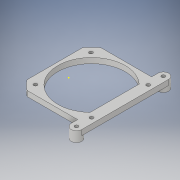
# Autodesk Inventor part: END
Saved by Autodesk Inventor 2019.4 (Build 234330000, 330)
## iProperties
Created: 2020-08-29
Part Number: END
Material: Generic
Document SubType Name: Modeling
Designer: craig
Density: 1 g/cm^3
Appearance: Default
Author: craig
## iProperties of the stored document _3DPrint.ipt
Created: 2020-08-29
Part Number: _3DPrint
Material: Generic
Document SubType Name: Modeling
Designer: craig
Density: 1 g/cm^3
Appearance: Default
Author: craig
Autodesk Inventor part; units mm, degrees
ref_plane "YZ Plane" through (0, 0, 0) normal (1, 0, 0) x (0, 1, 0)
ref_plane "XZ Plane" through (0, 0, 0) normal (0, 1, 0) x (-1, 0, 0)
ref_plane "XY Plane" through (0, 0, 0) normal (0, 0, 1) x (1, 0, 0)
sketch "Sketch1" plane through (0, 0, 0) normal (0, 1, 0) x (-1, 0, 0)
  line L0 (29, 24.5) -> (-29, 24.5) construction
  line L1 (-29, 24.5) -> (-29, -24.5) construction
  line L2 (-29, -24.5) -> (29, -24.5) construction
  line L3 (29, -24.5) -> (29, 24.5) construction
  line L4 (29, 24.5) -> (-29, -24.5) construction
  line L5 (-29, 24.5) -> (29, -24.5) construction
  circle A0 centre (29, 24.5) radius 1
  circle A1 centre (29, -24.5) radius 1
  circle A2 centre (-29, -24.5) radius 1
  circle A3 centre (-29, 24.5) radius 1
  circle A4 centre (29, 24.5) radius 3
  circle A5 centre (29, -24.5) radius 3
  circle A6 centre (-29, -24.5) radius 3
  circle A7 centre (-29, 24.5) radius 3
  point P0 (0, 0)
  dimension "d0" = 49
  dimension "d1" = 58
  dimension "d2" = 2
  dimension "d3" = 6
  constraints: 12 end point, 8 centre point, 8 coincident, 6 equal radius, 2 midpoint, 2 parallel, 1 horizontal, 1 perpendicular
  measures "d0" distance of L2.end L0.start
  measures "d1" distance of L0.start L0.end
  measures "d2" diameter of A0
  measures "d3" diameter of A4
extrude "Extrusion1" add sketch "Sketch1" along normal blind 5.8
sketch "Sketch2" plane through (-29, 5.8, 24.5) normal (0, 1, 0) x (1, 0, 0)
  line L0 (3, -0.001) -> (3, 48.999)
  line L1 (-3, 48.999) -> (-3, -0.001)
  circle A0 centre (0, 0) radius 1 projected
  line L2 (61, 0) -> (61, 49)
  line L3 (55, 49) -> (55, 0)
  circle A1 centre (58, 0) radius 1 projected
  circle A2 centre (0, 49) radius 1 projected
  circle A3 centre (58, 49) radius 1 projected
  line L4 (-3, -0.001) -> (-1, -0.001)
  line L5 (1, -0.001) -> (3, -0.001)
  line L6 (3, 48.999) -> (1, 48.999)
  line L7 (-1, 48.999) -> (-3, 48.999)
  line L8 (61, 49) -> (59, 49)
  line L9 (57, 49) -> (55, 49)
  line L10 (55, 0) -> (57, 0)
  line L11 (59, 0) -> (61, 0)
  point P0 (29, 24.5)
  dimension "d6" = 6
  dimension "d7" = 3
  dimension "d8" = 49
  dimension "d9" = 49
  dimension "d10" = 6
  dimension "d11" = 3
  constraints: 24 end point, 10 parallel, 8 point on circle, 4 horizontal, 4 perpendicular
  measures "d6" distance of L1.end L0.start
  measures "d7" distance from line of A0.centre L1
  measures "d8" distance of L1.start L1.end
  measures "d9" distance of L3.start L3.end
  measures "d10" distance of L3.end L2.start
  measures "d11" distance from line of A1.centre L3
extrude "Extrusion2" add sketch "Sketch2" against normal blind 3
sketch "Sketch3" plane through (-29, 2.8, 24.5) normal (0, -1, 0) x (1, 0, 0)
  circle A0 centre (0, -5) radius 2.5
  circle A1 centre (0, 0) radius 1 projected
  point P0 (29, -24.5)
  dimension "d14" = 5
  dimension "d15" = 5
  constraints: 1 centre point
  measures "d14" diameter of A0
  measures "d15" distance of A1.centre A0.centre
extrude "Extrusion3" cut sketch "Sketch3" against normal blind 2.8 contours A0
sketch "Sketch4" plane through (0, 5.8, 0) normal (0, 1, 0) x (1, 0, 0)
  circle A0 centre (29, -16) radius 1
  circle A1 centre (29, 16) radius 1
  circle A2 centre (29, -24.5) radius 1 projected
  point P0 (0, 0)
  dimension "d18" = 32
  dimension "d19" = 16
  dimension "d20" = 2
  dimension "d21" = 2
  dimension "d22" = 0
  constraints: 2 centre point, 1 vertical alignment
  measures "d18" distance of A1.centre A0.centre
  measures "d19" vertical distance of point (0, 0) A0.centre
  measures "d20" diameter of A0
  measures "d21" diameter of A1
  measures "d22" horizontal distance of A2.centre A0.centre
extrude "Extrusion4" cut sketch "Sketch4" against normal blind 2.8 contours A0 | A1
sketch "Sketch5" plane through (0, 5.8, 0) normal (0, 1, 0) x (1, 0, 0)
  line L0 (26, -24.5) -> (26, 24.5) projected
  circle A0 centre (-3, -15.6503) radius 0.9959
  circle A1 centre (29, -16) radius 1 projected
  arc A2 (-6, 0) -> (26, -13.8564) centre (13, 0) ccw
  arc A3 (-13, 0) -> (26, -22.5167) centre (13, 0) ccw
  line L1 (-13, 0) -> (-6, 0)
  point P0 (0, 0)
  dimension "d27" = 32
  dimension "d37" = 38
  dimension "d38" = 16
  dimension "d39" = 52
  constraints: 4 point on circle, 3 centre point, 2 end point, 2 point on line, 1 coincident
  measures "d27" horizontal distance of A1.centre A0.centre
  measures "d37" diameter of A2
  measures "d38" horizontal distance of A2.centre A0.centre
  measures "d39" diameter of A3
sketch "Sketch6" plane through (-29, 0, 24.5) normal (0, -1, 0) x (1, 0, 0)
  line L0 (-8.1916, 7.2928) -> (10.6769, 7.2928)
  line L1 (10.6769, 7.2928) -> (10.6769, -56.4019)
  line L2 (10.6769, -56.4019) -> (-8.1916, -56.4019)
  line L3 (-8.1916, -56.4019) -> (-8.1916, 7.2928)
  point P0 (29, -24.5)
  constraints: 8 end point, 2 parallel, 1 horizontal, 1 perpendicular
extrude "Extrusion6" cut sketch "Sketch6" against normal blind 6
sketch "Sketch7" plane through (29, 2.8, -24.5) normal (0, -1, 0) x (1, 0, 0)
  circle A0 centre (0, 0) radius 1 projected
  circle A1 centre (0, 49) radius 1 projected
  circle A2 centre (0, 8.5) radius 1 projected
  circle A3 centre (0, 40.5) radius 1 projected
  point P0 (-29, 24.5)
extrude "Extrusion7" cut sketch "Sketch7" along normal mid plane 10
sketch "Sketch8" plane through (-29, 2.8, 24.5) normal (0, -1, 0) x (1, 0, 0)
  point P0 (29, -24.5)
extrude "Extrusion8" add sketch "Sketch5" against normal blind 3 contours A3 L1 A2 L0
mirror "Mirror2" about plane through (-13, 5.8, 0) normal (0, 0, -1) of "Extrusion8"
sketch "Sketch9" plane through (0, 5.8, 0) normal (0, 1, 0) x (1, 0, 0)
  line L0 (-2.5176, -20.8616) -> (26, -20.8616)
  line L1 (26, -20.8616) -> (26, -22.5167)
  arc A0 (-2.5176, -20.8616) -> (26, -22.5167) centre (13, 0) ccw
  point P0 (0, 0)
  constraints: 4 end point, 2 point on circle, 1 centre point, 1 horizontal, 1 perpendicular
extrude "Extrusion9" cut sketch "Sketch9" against normal blind 3
mirror "Mirror3" about plane through (0, 0, 0) normal (0, 0, 1) of "Extrusion9"
sketch "Sketch10" plane through (-29, 2.8, 24.5) normal (0, -1, 0) x (1, 0, 0)
  line L0 (21.2476, -6.8926) -> (21.2476, -43.4948)
  line L1 (21.2476, -6.8926) -> (8.6589, -25.9252)
  line L2 (8.6589, -25.9252) -> (21.2476, -43.4948)
  point P0 (29, -24.5)
  constraints: 6 end point, 1 vertical
extrude "Extrusion10" cut sketch "Sketch10" against normal blind 3
equation "\"d21\" = d20"
body "Solid1"
